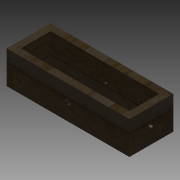
# Autodesk Inventor part: gyroWheelCradle01
Saved by Autodesk Inventor 2013 (Build 170138000, 138)
## iProperties
Created: 2013-02-23
Part Number: gyroWheelCradle01
Material: Wood (Maple)
Document SubType Name: Modeling
Designer: Nano
Density: 0.57 g/cm^3
Mass: 794.435 g
Surface Area: 1809.38 cm^2
Volume: 1393.75 cm^3
Author: Nano
Autodesk Inventor part; units mm, degrees
ref_plane "YZ Plane" through (0, 0, 0) normal (1, 0, 0) x (0, 1, 0)
ref_plane "XZ Plane" through (0, 0, 0) normal (0, 1, 0) x (-1, 0, 0)
ref_plane "XY Plane" through (0, 0, 0) normal (0, 0, 1) x (1, 0, 0)
sketch "Sketch1" plane through (0, 0, 0) normal (0, 1, 0) x (-1, 0, 0)
  line L0 (-166.6875, -59.5312) -> (166.6875, -59.5312)
  line L1 (166.6875, -59.5312) -> (166.6875, 59.5312)
  line L2 (166.6875, 59.5312) -> (-166.6875, 59.5312)
  line L3 (-166.6875, 59.5312) -> (-166.6875, -59.5312)
  line L4 (-166.6875, -59.5312) -> (166.6875, 59.5312) construction
  line L5 (166.6875, -59.5312) -> (-166.6875, 59.5312) construction
  point P0 (0, 0)
  point P1 (0, 0)
  dimension "d0" = 333.375
  dimension "d1" = 119.0625
  constraints: 12 end point, 2 midpoint, 2 parallel, 1 horizontal, 1 perpendicular
  measures "d0" distance of L2.end L1.end
  measures "d1" distance of L1.end L0.end
extrude "Extrusion1" add sketch "Sketch1" along normal blind 88.9
sketch "Sketch2" plane through (0, 88.9, 0) normal (0, 1, 0) x (1, 0, 0)
  line L0 (166.6875, 59.5312) -> (-166.6875, 59.5312) projected
  line L1 (-166.6875, 59.5312) -> (-166.6875, -59.5312) projected
  line L2 (-166.6875, -59.5312) -> (166.6875, -59.5312) projected
  line L3 (166.6875, -59.5312) -> (166.6875, 59.5312) projected
  line L4 (-147.6375, 40.4812) -> (147.6375, 40.4812)
  line L5 (147.6375, 40.4812) -> (147.6375, -40.4812)
  line L6 (147.6375, -40.4812) -> (-147.6375, -40.4813)
  line L7 (-147.6375, -40.4813) -> (-147.6375, 40.4812)
  point P0 (0, 0)
  dimension "d4" = 19.05
  dimension "d5" = 19.05
  dimension "d6" = 19.05
  dimension "d7" = 19.05
  constraints: 8 end point, 2 parallel, 1 horizontal, 1 perpendicular
  measures "d4" distance between parallel lines of L7 L1
  measures "d5" distance between parallel lines of L3 L5
  measures "d6" distance between parallel lines of L4 L0
  measures "d7" distance between parallel lines of L2 L6
extrude "Extrusion2" cut sketch "Sketch2" against normal through all contours L4 L5 L6 L7
sketch "Sketch3" plane through (166.6875, 0, -59.5312) normal (0, 0, -1) x (-1, 0, 0)
  line L0 (0, 88.9) -> (333.375, 0) construction
  line L1 (0, 0) -> (333.375, 88.9) construction
  point P0 (166.6875, 0)
  point P1 (166.6875, 44.45)
  constraints: 4 end point
hole "Hole1" at (0, 44.45, -59.5312) direction (0, 0, 1) diameter 12.7 end through all
sketch "Sketch4" plane through (166.6875, 0, 59.5312) normal (1, 0, 0) x (0, 0, -1)
  line L0 (0, 0) -> (119.0625, 88.9) construction
  line L1 (0, 88.9) -> (119.0625, 0) construction
  point P0 (59.5312, 0)
  point P1 (59.5312, 44.45)
  constraints: 4 end point
hole "Hole2" at (166.6875, 44.45, 0) direction (-1, 0, 0) diameter 12.7 end through all
equation "\"d5\" = d4"
equation "\"d6\" = d4"
equation "\"d7\" = d4"
body "Solid1"
